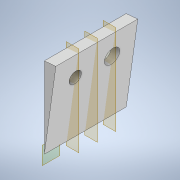
# Autodesk Inventor part: twoPipeCover
Saved by Autodesk Inventor 2021 (Build 250183000, 183)
## iProperties
Created: 2020-07-06
Part Number: twoPipeCover
Material: Generic
Document SubType Name: Modeling
Designer: robst
Density: 1 g/cm^3
Appearance: Default
Author: robst
Autodesk Inventor part; units mm, degrees
ref_plane "YZ Plane" through (0, 0, 0) normal (1, 0, 0) x (0, 1, 0)
ref_plane "XZ Plane" through (0, 0, 0) normal (0, 1, 0) x (-1, 0, 0)
sketch "Sketch1" plane through (0, 0, 0) normal (0, 0, 1) x (1, 0, 0)
  line L0 (0, 0) -> (14.2789, 101.6)
  line L1 (14.2789, 101.6) -> (0, 101.6)
  line L2 (0, 101.6) -> (0, 0)
  dimension "d0" = 101.6
  dimension "d1" = 8
  dimension "d2" = 14.279
  constraints: 6 end point, 1 horizontal, 1 vertical
  measures "d0" distance from line of L0.start L1
  measures "d1" angle of L0 L2
  measures "d2" distance of L0.end L1.end
extrude "Extrusion1" add sketch "Sketch1" along normal mid plane 101.6
ref_plane "Work Plane2" through (0, 0, 42.3872) normal (-1, 0, 0) x (0, 0, 1)
sketch "Sketch7" plane through (0, 0, 0) normal (0, 0, 1) x (1, 0, 0)
  line L0 (0, 101.6) -> (14.2789, 101.6) projected
  line L1 (0, 0) -> (14.2789, 101.6) projected
  line L2 (0, 101.6) -> (0, 0) projected
  line L3 (14.2789, 101.6) -> (0, 101.6) projected
  line L4 (14.2789, 101.6) -> (0, 100.3508)
  line L5 (0, 100.3508) -> (0, 101.6)
  line L6 (0, 101.6) -> (14.2789, 101.6)
  dimension "d27" = 5
  constraints: 6 end point, 1 collinear, 1 perpendicular, 1 point on line
  measures "d27" angle of L0 L4
extrude "Extrusion6" cut sketch "Sketch7" along normal through all both and the other way through all contours L0 L4 L2
sketch "Sketch6" plane through (0, 0, 42.3872) normal (-1, 0, 0) x (0, 0, 1)
  line L0 (-84.1061, 73.66) -> (0, 73.66) construction
  line L1 (0, 101.6) -> (0, 0) construction
  line L2 (-84.7743, 101.6) -> (0, 101.6) construction
  circle A0 centre (-65.2472, 73.66) radius 9.525
  circle A1 centre (-19.5272, 73.66) radius 7.62
  line L3 (-42.3872, 121.92) -> (-42.3872, -20.32) projected
  point P0 (-42.3872, 0)
  dimension "d18" = 27.94
  dimension "d19" = 19.05
  dimension "d20" = 15.24
  dimension "d21" = 22.86
  dimension "d22" = 22.86
  dimension "d23" = 45.72
  constraints: 3 point on line, 2 centre point, 2 end point, 1 horizontal
  measures "d18" distance between parallel lines of L0 L2
  measures "d19" diameter of A0
  measures "d20" diameter of A1
  measures "d21" distance from line of L3 A0.centre
  measures "d22" distance from line of A1.centre L3
  measures "d23" distance of A1.centre A0.centre
extrude "Extrusion5" cut sketch "Sketch6" against normal through all
ref_plane "Work Plane3" through (0, 0, 22.86) normal (0, 0, 1) x (1, 0, 0)
ref_plane "Work Plane4" through (0, 0, -22.86) normal (0, 0, 1) x (1, 0, 0)
body "Solid1"
